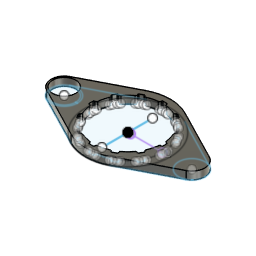
桶盖扳手 (Autodesk Fusion 360 design; units mm, degrees)
Autodesk Fusion 360 part; units mm, degrees
note: some values were not read from the file. Set by a fixed rule: which sketch regions a step uses.
sketch "草图1" plane through (0, 0, 0) normal (0, 0, 1) x (1, 0, 0)
  line L0 (0, 16) -> (0, -17)
  circle A0 centre (0, 0) radius 27.5
  line L1 (24, 1.25) -> (24, -1.25)
  line L2 (-23.5, 1.75) -> (-23.3385, 1.75)
  line L3 (23.3385, 1.75) -> (23.5, 1.75)
  line L4 (23.5, -1.75) -> (23.3385, -1.75)
  line L5 (-23.3385, -1.75) -> (-23.5, -1.75)
  line L6 (21.2266, 10.2345) -> (21.0868, 10.1537)
  line L7 (20.1596, 13.0825) -> (21.4096, 10.9175)
  line L8 (19.3368, 13.1848) -> (19.4766, 13.2655)
  line L9 (13.2655, 19.4766) -> (13.1848, 19.3368)
  line L10 (10.9175, 21.4096) -> (13.0825, 20.1596)
  line L11 (10.1537, 21.0868) -> (10.2345, 21.2266)
  line L12 (1.75, 23.5) -> (1.75, 23.3385)
  line L13 (-1.75, 23.3385) -> (-1.75, 23.5)
  line L14 (-10.2345, 21.2266) -> (-10.1537, 21.0868)
  line L15 (-13.0825, 20.1596) -> (-10.9175, 21.4096)
  line L16 (-13.1848, 19.3368) -> (-13.2655, 19.4766)
  line L17 (-19.4766, 13.2655) -> (-19.3368, 13.1848)
  line L18 (-21.0868, 10.1537) -> (-21.2266, 10.2345)
  line L19 (-23.5, 1.75) -> (-23.3385, 1.75)
  line L20 (-23.3385, -1.75) -> (-23.5, -1.75)
  line L21 (-21.2266, -10.2345) -> (-21.0868, -10.1537)
  line L22 (-19.3368, -13.1848) -> (-19.4766, -13.2655)
  line L23 (-13.2655, -19.4766) -> (-13.1848, -19.3368)
  line L24 (-10.1537, -21.0868) -> (-10.2345, -21.2266)
  line L25 (-1.75, -23.5) -> (-1.75, -23.3385)
  line L26 (1.25, -24) -> (-1.25, -24)
  line L27 (1.75, -23.3385) -> (1.75, -23.5)
  line L28 (10.2345, -21.2266) -> (10.1537, -21.0868)
  line L29 (13.1848, -19.3368) -> (13.2655, -19.4766)
  line L30 (19.4766, -13.2655) -> (19.3368, -13.1848)
  line L31 (21.0868, -10.1537) -> (21.2266, -10.2345)
  arc A1 (20.6682, -8.8925) -> (22.3454, -2.633) centre (0, 0) ccw
  arc A2 (13.4529, -18.0352) -> (18.0352, -13.4529) centre (0, 0) ccw
  arc A3 (2.633, -22.3454) -> (8.8925, -20.6682) centre (0, 0) ccw
  arc A4 (-8.8925, -20.6682) -> (-2.633, -22.3454) centre (0, 0) ccw
  arc A5 (-22.3454, -2.633) -> (-20.6682, -8.8925) centre (0, 0) ccw
  arc A6 (-18.0352, -13.4529) -> (-13.4529, -18.0352) centre (0, 0) ccw
  arc A7 (22.3454, 2.633) -> (20.6682, 8.8925) centre (0, 0) ccw
  arc A8 (18.0352, 13.4529) -> (13.4529, 18.0352) centre (0, 0) ccw
  arc A9 (8.8925, 20.6682) -> (2.633, 22.3454) centre (0, 0) ccw
  arc A10 (-2.633, 22.3454) -> (-8.8925, 20.6682) centre (0, 0) ccw
  arc A11 (-13.4529, 18.0352) -> (-18.0352, 13.4529) centre (0, 0) ccw
  arc A12 (-20.6682, 8.8925) -> (-22.3454, 2.633) centre (0, 0) ccw
  line L32 (1.75, 0) -> (22.5, 0)
  arc A13 (23.3385, -1.75) -> (22.3454, -2.633) centre (23.3385, -2.75) ccw
  arc A14 (22.3454, 2.633) -> (23.3385, 1.75) centre (23.3385, 2.75) ccw
  arc A15 (24, 1.25) -> (23.5, 1.75) centre (23.5, 1.25) ccw
  arc A16 (23.5, -1.75) -> (24, -1.25) centre (23.5, -1.25) ccw
  arc A17 (18.0352, 13.4529) -> (19.3368, 13.1848) centre (18.8368, 14.0508) ccw
  arc A18 (20.1596, 13.0825) -> (19.4766, 13.2655) centre (19.7266, 12.8325) ccw
  line L33 (20.1596, 13.0825) -> (21.4096, 10.9175)
  arc A19 (21.2266, 10.2345) -> (21.4096, 10.9175) centre (20.9766, 10.6675) ccw
  arc A20 (21.0868, 10.1537) -> (20.6682, 8.8925) centre (21.5868, 9.2877) ccw
  arc A21 (8.8925, 20.6682) -> (10.1537, 21.0868) centre (9.2877, 21.5868) ccw
  arc A22 (10.9175, 21.4096) -> (10.2345, 21.2266) centre (10.6675, 20.9766) ccw
  arc A23 (13.2655, 19.4766) -> (13.0825, 20.1596) centre (12.8325, 19.7266) ccw
  arc A24 (13.1848, 19.3368) -> (13.4529, 18.0352) centre (14.0508, 18.8368) ccw
  arc A25 (-2.633, 22.3454) -> (-1.75, 23.3385) centre (-2.75, 23.3385) ccw
  arc A26 (-1.25, 24) -> (-1.75, 23.5) centre (-1.25, 23.5) ccw
  line L34 (-1.25, 24) -> (1.25, 24)
  arc A27 (1.75, 23.5) -> (1.25, 24) centre (1.25, 23.5) ccw
  arc A28 (1.75, 23.3385) -> (2.633, 22.3454) centre (2.75, 23.3385) ccw
  arc A29 (-13.4529, 18.0352) -> (-13.1848, 19.3368) centre (-14.0508, 18.8368) ccw
  arc A30 (-13.0825, 20.1596) -> (-13.2655, 19.4766) centre (-12.8325, 19.7266) ccw
  arc A31 (-10.2345, 21.2266) -> (-10.9175, 21.4096) centre (-10.6675, 20.9766) ccw
  arc A32 (-10.1537, 21.0868) -> (-8.8925, 20.6682) centre (-9.2877, 21.5868) ccw
  arc A33 (-20.6682, 8.8925) -> (-21.0868, 10.1537) centre (-21.5868, 9.2877) ccw
  arc A34 (-21.4096, 10.9175) -> (-21.2266, 10.2345) centre (-20.9766, 10.6675) ccw
  line L35 (-21.4096, 10.9175) -> (-20.1596, 13.0825)
  arc A35 (-19.4766, 13.2655) -> (-20.1596, 13.0825) centre (-19.7266, 12.8325) ccw
  arc A36 (-19.3368, 13.1848) -> (-18.0352, 13.4529) centre (-18.8368, 14.0508) ccw
  arc A37 (-22.3454, -2.633) -> (-23.3385, -1.75) centre (-23.3385, -2.75) ccw
  arc A38 (-24, -1.25) -> (-23.5, -1.75) centre (-23.5, -1.25) ccw
  line L36 (-24, -1.25) -> (-24, 1.25)
  arc A39 (-23.5, 1.75) -> (-24, 1.25) centre (-23.5, 1.25) ccw
  arc A40 (-23.3385, 1.75) -> (-22.3454, 2.633) centre (-23.3385, 2.75) ccw
  arc A41 (-18.0352, -13.4529) -> (-19.3368, -13.1848) centre (-18.8368, -14.0508) ccw
  arc A42 (-20.1596, -13.0825) -> (-19.4766, -13.2655) centre (-19.7266, -12.8325) ccw
  line L37 (-20.1596, -13.0825) -> (-21.4096, -10.9175)
  arc A43 (-21.2266, -10.2345) -> (-21.4096, -10.9175) centre (-20.9766, -10.6675) ccw
  arc A44 (-21.0868, -10.1537) -> (-20.6682, -8.8925) centre (-21.5868, -9.2877) ccw
  arc A45 (-8.8925, -20.6682) -> (-10.1537, -21.0868) centre (-9.2877, -21.5868) ccw
  arc A46 (-10.9175, -21.4096) -> (-10.2345, -21.2266) centre (-10.6675, -20.9766) ccw
  line L38 (-10.9175, -21.4096) -> (-13.0825, -20.1596)
  arc A47 (-13.2655, -19.4766) -> (-13.0825, -20.1596) centre (-12.8325, -19.7266) ccw
  arc A48 (-13.1848, -19.3368) -> (-13.4529, -18.0352) centre (-14.0508, -18.8368) ccw
  arc A49 (2.633, -22.3454) -> (1.75, -23.3385) centre (2.75, -23.3385) ccw
  arc A50 (1.25, -24) -> (1.75, -23.5) centre (1.25, -23.5) ccw
  arc A51 (-1.75, -23.5) -> (-1.25, -24) centre (-1.25, -23.5) ccw
  arc A52 (-1.75, -23.3385) -> (-2.633, -22.3454) centre (-2.75, -23.3385) ccw
  arc A53 (13.4529, -18.0352) -> (13.1848, -19.3368) centre (14.0508, -18.8368) ccw
  arc A54 (13.0825, -20.1596) -> (13.2655, -19.4766) centre (12.8325, -19.7266) ccw
  line L39 (13.0825, -20.1596) -> (10.9175, -21.4096)
  arc A55 (10.2345, -21.2266) -> (10.9175, -21.4096) centre (10.6675, -20.9766) ccw
  arc A56 (10.1537, -21.0868) -> (8.8925, -20.6682) centre (9.2877, -21.5868) ccw
  arc A57 (20.6682, -8.8925) -> (21.0868, -10.1537) centre (21.5868, -9.2877) ccw
  arc A58 (21.4096, -10.9175) -> (21.2266, -10.2345) centre (20.9766, -10.6675) ccw
  line L40 (21.4096, -10.9175) -> (20.1596, -13.0825)
  arc A59 (19.4766, -13.2655) -> (20.1596, -13.0825) centre (19.7266, -12.8325) ccw
  arc A60 (19.3368, -13.1848) -> (18.0352, -13.4529) centre (18.8368, -14.0508) ccw
  circle A61 centre (-41.5, -0.0111) radius 8.5
  circle A62 centre (41.5, -0.0111) radius 8.5
  line L41 (0, 16) -> (0, -17)
  line L42 (-45.3936, 7.5447) -> (-12.5969, 24.4452)
  line L43 (45.3936, 7.5447) -> (12.5969, 24.4452)
  line L44 (45.3895, -7.5689) -> (12.5838, -24.4519)
  line L45 (-45.3895, -7.5689) -> (-12.5838, -24.4519)
  circle A63 centre (-41.5, -0.0111) radius 7.5
  point P0 (24, 1.75)
  dimension "d1" = 45
  dimension "d2" = 55
  dimension "d38" = 1
  dimension "d39" = 1
  dimension "d40" = 0.5
  dimension "d41" = 0.5
  dimension "d43" = 360
  dimension "d55" = 17
  dimension "d56" = 41.5
  dimension "d59" = 15
  constraint coincident A0.centre L0
  constraint coincident A0.centre A1.centre
  constraint collinear L4 L5
  constraint concentric A5 A7
  constraint concentric A1 A5
  constraint concentric A2 A5
  constraint concentric A3 A5
  constraint concentric A4 A5
  constraint concentric A5 A6
  constraint concentric A7 A8
  constraint concentric A8 A9
  constraint concentric A9 A10
  constraint concentric A10 A11
  constraint concentric A11 A12
  constraint tangent L4 A13
  constraint tangent A1 A13
  constraint tangent L3 A14
  constraint tangent A7 A14
  constraint coincident P0 L1
  constraint coincident P0 L3
  constraint tangent L1 A15
  constraint tangent L3 A15
  constraint tangent L1 A16
  constraint tangent L4 A16
  constraint symmetric L41.start L0 L0.start
  constraint symmetric L41.end L0 L0.end
  constraint symmetric L0 A61 A62
  constraint coincident A61 L42.start
  constraint coincident A62 L43.start
  constraint coincident A0 L43.end
  constraint tangent A0 L43
  constraint coincident A62 L44.start
  constraint coincident A0 L44.end
  constraint tangent A0 L44
  constraint coincident A61 L45.start
  constraint coincident A0 L45.end
  constraint tangent A0 L45
  constraint coincident A0 L42.end
  constraint tangent A0 L42
  constraint tangent A62 L43
  constraint tangent A62 L44
  constraint tangent A61 L45
  constraint tangent A61 L42
  constraint concentric A61 A63
  measures "d1" diameter of A7
  measures "d2" diameter of A0
  measures "d38" radius of A13
  measures "d39" radius of A14
  measures "d40" radius of A15
  measures "d41" radius of A16
  measures "d55" diameter of A61
  measures "d56" horizontal distance of A0.centre A61.centre
  measures "d59" diameter of A63
extrude "拉伸6" add sketch "草图1" along normal blind 5
